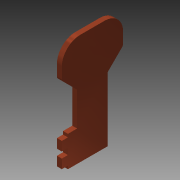
# Autodesk Inventor part: Key
Saved by Autodesk Inventor 2014 SP1 (Build 180222100, 222)
## iProperties
Created: 2016-06-11
Part Number: Key
Material: Copper
Document SubType Name: Sheet Metal
Designer: Tyler
Density: 8.94 g/cm^3
Sheet Metal Rule: Default_mm
Appearance: Copper - Satin
Author: Tyler
Autodesk Inventor part; units mm, degrees
ref_plane "YZ Plane" through (0, 0, 0) normal (1, 0, 0) x (0, 1, 0)
ref_plane "XZ Plane" through (0, 0, 0) normal (0, 1, 0) x (-1, 0, 0)
ref_plane "XY Plane" through (0, 0, 0) normal (0, 0, 1) x (1, 0, 0)
sketch "Sketch2" plane through (0, 0, 0) normal (-1, 0, 0) x (0, 0, 1)
  line L0 (0, 10) -> (0, 0)
  line L1 (0, 0) -> (5, 0)
  line L2 (10.4142, -5) -> (14, -5)
  line L3 (0, 10) -> (-16, 10)
  line L4 (-16, 10) -> (-16, -3)
  line L5 (-6, -3) -> (-6, 0)
  line L6 (-6, 0) -> (0, 0)
  line L7 (-15, -3) -> (-15, -5)
  line L8 (-15, -5) -> (-12, -5)
  line L9 (-12, -5) -> (-12, -3)
  line L10 (-10, -3) -> (-10, -5)
  line L11 (-10, -5) -> (-7, -5)
  line L12 (-7, -5) -> (-7, -3)
  line L13 (-7, -3) -> (-6, -3)
  line L14 (-16, -3) -> (-15, -3)
  line L15 (-12, -3) -> (-10, -3)
  dimension "d10" = 2
  dimension "d11" = 3
  dimension "d12" = 3
  dimension "d13" = 1
  dimension "d14" = 1
  dimension "d15" = 2
  dimension "d16" = 2
  dimension "d17" = 3
  dimension "d18" = 6
  measures "d10" distance between parallel lines of L9 L10
  measures "d11" distance of L10.end L11.end
  measures "d12" distance of L7.end L8.end
  measures "d13" distance between parallel lines of L4 L7
  measures "d14" distance between parallel lines of L12 L5
  measures "d15" distance of L11.end L12.end
  measures "d16" distance of L8.end L9.end
  measures "d17" distance between parallel lines of L13 L6
  measures "d18" distance between parallel lines of L0 L5
sketch "Sketch1" plane through (0, 0, 0) normal (1, 0, 0) x (0, 1, 0)
  line L0 (0, 0) -> (0, 5)
  line L1 (0, 5) -> (-5, 10)
  line L2 (-5, 10) -> (15, 10) construction
  line L3 (15, 10) -> (10, 5)
  line L4 (10, 5) -> (10, 0)
  line L5 (10, 0) -> (0, 0)
  line L6 (-5, 10) -> (-5, 20)
  line L7 (-5, 20) -> (15, 20)
  line L8 (15, 20) -> (15, 10)
  dimension "d0" = 10
  dimension "d1" = 45
  dimension "d2" = 45
  dimension "d3" = 5
  dimension "d4" = 5
  dimension "d5" = 10
  dimension "d8" = 10
  measures "d0" distance between parallel lines of L0 L4
  measures "d1" angle of L2 L3
  measures "d2" angle of L2 L1
  measures "d3" distance from line of L2.end L4
  measures "d4" distance from line of L0 L1.end
  measures "d5" distance between parallel lines of L5 L2
  measures "d8" distance of L7.end L2.end
extrude "Plate1" add sketch "Sketch1" along normal blind 1.6
fillet "Corner Round1" radius 1 2 edges at (0.8, 15, 10) (0.8, -5, 10)
fillet "Corner Round2" radius 6 2 edges at (0.8, 15, 20) (0.8, -5, 20)
sheet face with bend "Face2" sketch "Sketch2" thickness 1.6 toward (1, 0, 0) bend radius 1.6 relief straight relief width 1.6 relief depth 0.8
bend "Bend1"
equation "\"d19\" = BendRadius"
equation "\"d20\" = BendReliefWidth"
equation "\"d22\" = MinimumRemnant"
equation "\"d21\" = BendReliefDepth"
equation "\"d23\" = BendRadius"
equation "\"BendRadius\" = Thickness"
equation "\"BendReliefWidth\" = Thickness"
equation "\"BendReliefDepth\" = 0.5 * Thickness"
equation "\"CornerReliefSize\" = 4 * Thickness"
equation "\"MinimumRemnant\" = 2 * Thickness"
equation "\"TransitionRadius\" = BendRadius"
equation "\"JacobiRadiusSize\" = BendRadius"
equation "\"GapSize\" = Thickness"
equation "\"d6\" = BendRadius"
equation "\"Thickness\" = 1.6"
body "Solid1"
